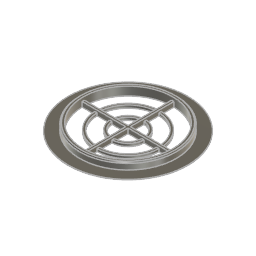
Garbage Disposal Shot Glass Saver (Autodesk Fusion 360 design; units mm, degrees)
Autodesk Fusion 360 part; units mm, degrees
sketch "Sketch1" plane through (0, 0, 0) normal (0, 0, 1) x (1, 0, 0)
  circle A0 centre (0, 0) radius 42
  circle A1 centre (0, 0) radius 52
  circle A2 centre (0, 0) radius 39
  dimension "d1" = 84
  dimension "d6" = 10
  dimension "d7" = 3
  constraint coincident A0.centre A1.centre
  constraint concentric A0 A1
  constraint concentric A1 A2
  measures "d1" diameter of A0
  measures "d6" distance of A0 A1
  measures "d7" distance of A0 A2
extrude "Extrude1" add sketch "Sketch1" along normal blind 2 contours A1 makes body 1
extrude "Extrude2" add sketch "Sketch1" along normal blind 8 contours A0 bodies 1
sketch "Sketch2" plane through (0, 0, 0) normal (0, 0, 1) x (1, 0, 0)
  circle A0 centre (0, 0) radius 39
  circle A1 centre (0, 0) radius 13
  circle A2 centre (0, 0) radius 26
  circle A3 centre (0, 0) radius 15
  circle A4 centre (0, 0) radius 28
  line L0 (-1, 38.9872) -> (-1, 0)
  line L1 (0, 1.75) -> (0, 22.5) construction
  line L2 (1, 38.9872) -> (1, 0)
  line L3 (1, 0) -> (-1, 0)
  dimension "d10" = 2
  dimension "d11" = 2
  dimension "d12" = 78
  dimension "d13" = 52
  dimension "d14" = 26
  dimension "d15" = 2
  constraint concentric A0 A1
  constraint concentric A0 A2
  constraint coincident A0 L0.start
  constraint vertical L0
  constraint symmetric L0.start L1 L2.start
  constraint symmetric L0.end L1 L2.end
  constraint horizontal A0.centre L0.end
  measures "d12" diameter of A0
  measures "d13" diameter of A2
  measures "d14" diameter of A1
  measures "d15" distance of L0 L2
extrude "Extrude3" add sketch "Sketch2" along normal blind 3 separate body contours A2 A4 L0 L2 | A1 A3 L0 L2 picked at (-2.3548, 27.167) picked at (-1.7411, 14.1926) makes body 2 at (-2.2847, 12.7977, 1) makes body 3 at (16.8382, -22.3713, 2)
extrude "Extrude4" add sketch "Sketch2" along normal blind 5 separate body contours A0 A4 L0 L2 | A2 A4 L0 L2 | A2 A3 L0 L2 | A1 A3 L0 L2 | A1 L0 L2 L3 picked at (0.7778, 31.6558) picked at (0.7778, 26.6536) picked at (-0.7779, 18.6479) picked at (0.7779, 13.6413) picked at (-0.1112, 4.3319) makes body 4
pattern_circular "C-Pattern1" count 4 over 360 about axis through (0, 0, 1.75) along (0, 0, 1) of "Extrude4" makes body 5 at (-8.641, -0.3333, 0) makes body 6 at (0.3333, -8.641, 0) makes body 7 at (8.641, 0.3333, 0)
chamfer "Chamfer1" distance 1.6 distance2 2.4 1 edges at (-48.481, -18.804, 0) measured on face at (51.9354, -2.592, 1.3333) on bodies 1
combine "Combine1" operation add target body 1 tool bodies 2 3 4 6 7 5
chamfer "Chamfer3" distance 0.6 angle 45 1 faces at (13.5849, 43.9212, 0) on bodies 1
chamfer "Chamfer4" distance 1 angle 45 1 edges at (-39.1577, -15.1878, 8) on bodies 1
chamfer "Chamfer2" [rolled back] distance 0.6
equation "d13 = d12 / 3 * 2"
equation "d14 = d12 / 3"
named bodies: "Garbage Disposal Shot Glass Saver"
